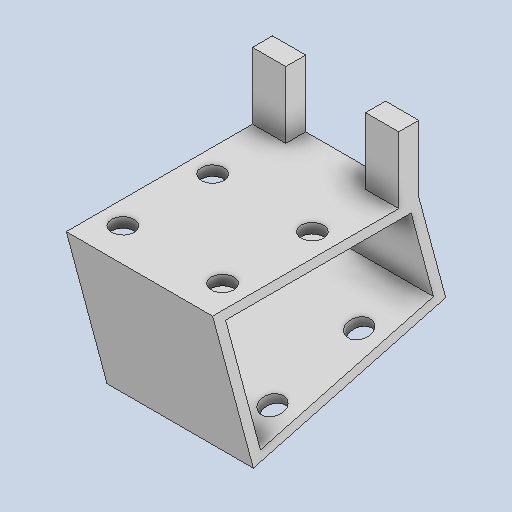
# Autodesk Inventor part: Ramp
Saved by Autodesk Inventor 2025.1 (Build 291241020, 241B)
## iProperties
Created: 2024-08-27
Part Number: Ramp
Material: Generic
Document SubType Name: Modeling
Designer: znghi
Density: 1 g/cm^3
Appearance: Default
Description: Ramp
Author: znghi
Autodesk Inventor part; units mm, degrees
note: some values were not read from the file. Chosen so that the rebuilt part matches the saved one: direction of "Hole2"; direction of "Hole3".
ref_plane "YZ Plane" through (0, 0, 0) normal (1, 0, 0) x (0, 1, 0)
ref_plane "XZ Plane" through (0, 0, 0) normal (0, 1, 0) x (-1, 0, 0)
ref_plane "XY Plane" through (0, 0, 0) normal (0, 0, 1) x (1, 0, 0)
sketch "Sketch1" plane through (0, 0, 0) normal (0, 1, 0) x (-1, 0, 0)
  line L0 (15, 13.5) -> (15, -13.5)
  line L1 (15, -13.5) -> (-15, -13.5)
  line L2 (-15, -13.5) -> (-15, 13.5)
  line L3 (-15, 13.5) -> (15, 13.5)
  point P0 (0, -13.5)
  point P1 (-15, 0)
  dimension "d2" = 27
  dimension "d3" = 30
  constraints: 8 end point, 2 midpoint, 2 perpendicular, 1 horizontal, 1 vertical
  measures "d2" distance of L0.start L0.end
  measures "d3" distance of L0.end L1.end
extrude "Extrusion1" [suppressed]
sketch "Sketch4" plane through (0, 0, 0) normal (1, 0, 0) x (0, 1, 0)
  line L0 (-18.1177, -21.5508) -> (-25.8677, 7.3726)
  line L1 (0, 13.5) -> (-3, 13.5) projected
  line L2 (-17.057, -19.7137) -> (-4.5, -16.349)
  line L3 (-4.5, 11.5452) -> (-24.0306, 6.312)
  line L4 (-3, -17.5) -> (-3, 13.5)
  line L5 (-24.0306, 6.312) -> (-17.057, -19.7137)
  line L6 (-4.5, -16.349) -> (-4.5, 11.5452)
  line L7 (-3, -13.5) -> (-3, 13.5) projected
  line L8 (-3, 13.5) -> (-25.8677, 7.3726)
  line L9 (-3, -17.5) -> (-18.1177, -21.5508)
  point P0 (0, 0)
  point P1 (-51.8403, 80.9842)
  point P2 (-3, 0)
  point P3 (-3, 0)
  point P4 (-3, 0)
  point P5 (-14.2653, 8.9286)
  point P6 (-10.5588, -19.5254)
  dimension "d50" = 1.5
  dimension "d57" = 1.5
  dimension "d59" = 1.5
  dimension "d60" = 1.5
  dimension "d62" = 4
  dimension "d63" = 15
  dimension "d64" = 13
  constraints: 14 end point, 3 coincident, 3 midpoint, 3 parallel, 1 perpendicular, 1 point on line, 6 other
  measures "d50" distance between parallel lines of L0 L5
  measures "d57" distance from line of L4 L6.end
  measures "d59" distance from line of L8 point (-14.265, 8.929)
  measures "d60" distance from line of point (-10.559, -19.525) L2
  measures "d62" distance of L4.start L7.start
  measures "d63" angle of L6 L5
  measures "d64" distance of L5.end L6.start
extrude "Extrusion3" add sketch "Sketch4" along normal mid plane 22
sketch "Sketch5" plane through (11, 0, 0) normal (1, 0, 0) x (0, 0, -1)
  line L0 (17.5, -3) -> (-13.5, -3) projected
  line L1 (14.5, -3) -> (17.5, -3)
  line L2 (17.5, -3) -> (17.5, 7)
  line L3 (17.5, 7) -> (14.5, 7)
  line L4 (14.5, 7) -> (14.5, -3)
  point P0 (0, 0)
  point P1 (13.5, -3)
  dimension "d67" = 3
  dimension "d68" = 10
  constraints: 8 end point, 2 parallel, 1 horizontal, 1 perpendicular, 1 point on line
  measures "d67" distance of L2.end L3.end
  measures "d68" distance of L0.start L2.end
extrude "Extrusion4" add sketch "Sketch5" against normal blind 5
mirror "Mirror1" about plane through (0, 0, 0) normal (1, 0, 0) of "Extrusion4"
sketch "Sketch6" plane through (0, -3, 0) normal (0, 1, 0) x (1, 0, 0)
  line L0 (15, 13.5) -> (15, -13.5) projected
  line L1 (11, -13.5) -> (-11, -13.5) projected
  line L2 (-11, 13.5) -> (11, 13.5) projected
  point P0 (0, 0)
  point P1 (-7.5, 5)
  point P2 (7.5, 5)
  point P3 (7.5, -8.5)
  point P4 (-7.5, -8.5)
  dimension "d71" = 15
  dimension "d72" = 13.5
  dimension "d73" = 7.5
  dimension "d74" = 5
  dimension "d75" = 8.5
  constraints: 2 vertical alignment, 1 horizontal alignment
  measures "d71" distance of point (7.5, 5) point (-7.5, 5)
  measures "d72" distance of point (7.5, 5) point (7.5, -8.5)
  measures "d73" distance from line of L0 point (7.5, 5)
  measures "d74" distance from line of L1 point (7.5, -8.5)
  measures "d75" distance from line of L2 point (-7.5, 5)
hole "Hole2" at (-7.5, -3, -5) at (7.5, -3, -5) at (7.5, -3, 8.5) at (-7.5, -3, 8.5) direction (0, -1, 0) diameter 3.4 depth 1.5
sketch "Sketch7" plane through (-11, -24.0306, 6.312) normal (0, 0.9659258, 0.258819) x (1, 0, 0)
  line L0 (22, -1.5) -> (0, -1.5) projected
  line L1 (22, -1.5) -> (22, 28.4437) projected
  point P0 (11, 12.3165)
  point P1 (3.5, 19)
  point P2 (18.5, 19)
  point P3 (18.5, 5.5)
  point P4 (3.5, 5.5)
  dimension "d83" = 15
  dimension "d84" = 13.5
  dimension "d88" = 7
  dimension "d89" = 3.5
  constraints: 2 horizontal alignment, 2 vertical alignment
  measures "d83" distance of point (18.5, 19) point (3.5, 19)
  measures "d84" distance of point (18.5, 19) point (18.5, 5.5)
  measures "d88" distance from line of L0 point (18.5, 5.5)
  measures "d89" distance from line of L1 point (18.5, 19)
hole "Hole3" at (-7.5, -22.6071, 0.9994) at (7.5, -22.6071, 0.9994) at (7.5, -19.113, -12.0406) at (-7.5, -19.113, -12.0406) direction (0, -0.9659258, -0.258819) diameter 3.4 depth 1.5
body "Solid1"
